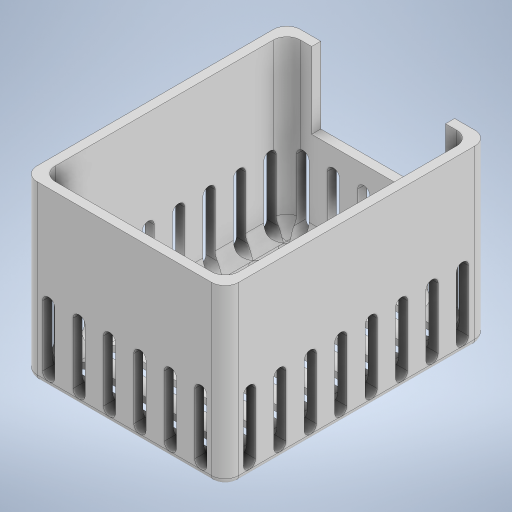
# Autodesk Inventor part: ProtectiveCase
Saved by Autodesk Inventor 2023 (Build 270158000, 158)
## iProperties
Created: 2024-02-01
Part Number: ProtectiveCase
Material: Generic
Document SubType Name: Modeling
Designer: Daniil
Density: 1 g/cm^3
Appearance: Default
Author: Daniil
Autodesk Inventor part; units mm, degrees
ref_plane "YZ Plane" through (0, 0, 0) normal (1, 0, 0) x (0, 1, 0)
ref_plane "XZ Plane" through (0, 0, 0) normal (0, 1, 0) x (-1, 0, 0)
ref_plane "XY Plane" through (0, 0, 0) normal (0, 0, 1) x (1, 0, 0)
sketch "Sketch1" plane through (0, 0, 0) normal (0, 1, 0) x (-1, 0, 0)
  line L0 (0, 0) -> (66.3, 0)
  line L1 (66.3, 0) -> (66.3, -86.6)
  line L2 (66.3, -86.6) -> (0, -86.6)
  line L3 (0, -86.6) -> (0, 0)
  line L4 (63.3, -3) -> (3, -3)
  line L5 (3, -3) -> (3, -83.6)
  line L6 (3, -83.6) -> (63.3, -83.6)
  line L7 (63.3, -83.6) -> (63.3, -3)
  dimension "d0" = 80.6
  dimension "d1" = 60.3
  dimension "d2" = 3
  dimension "d3" = 3
  dimension "d4" = 3
  dimension "d5" = 3
  constraints: 16 end point, 4 parallel, 2 horizontal, 2 perpendicular
  measures "d0" distance between parallel lines of L6 L4
  measures "d1" distance between parallel lines of L5 L7
  measures "d2" distance between parallel lines of L4 L0
  measures "d3" distance between parallel lines of L3 L5
  measures "d4" distance between parallel lines of L1 L7
  measures "d5" distance between parallel lines of L2 L6
extrude "Extrusion1" add sketch "Sketch1" along normal blind 57
sketch "Sketch2" plane through (0, 0, -86.6) normal (0, 0, -1) x (-1, 0, 0)
  line L0 (0, 0) -> (66.3, 0) projected
  line L1 (66.3, 0) -> (66.3, 57) projected
  line L2 (0, 57) -> (66.3, 57) projected
  line L3 (0, 0) -> (0, 57) projected
  line L4 (63.3, 57) -> (3, 57) construction
  line L5 (33.15, 57) -> (33.15, 0) construction
  line L6 (11.15, 57) -> (55.15, 57)
  line L7 (55.15, 57) -> (55.15, 35)
  line L8 (55.15, 35) -> (11.15, 35)
  line L9 (11.15, 35) -> (11.15, 57)
  point P0 (0, 0)
  dimension "d8" = 44
  dimension "d9" = 22
  constraints: 10 end point, 2 midpoint, 2 parallel, 1 horizontal, 1 perpendicular, 1 point on line, 1 other
  measures "d8" distance between parallel lines of L7 L9
  measures "d9" distance between parallel lines of L8 L2
extrude "Extrusion2" cut sketch "Sketch2" against normal blind 57 contours L2 L7 L8 L9
fillet "Fillet1" radius 4.5 8 edges at (-3, 28.5, -3) (-63.3, 28.5, -3) (-63.3, 28.5, -83.6) (-3, 28.5, -83.6) (0, 28.5, -86.6) (-66.3, 28.5, -86.6) (-66.3, 28.5, 0) (0, 28.5, 0)
sketch "Sketch3" plane through (0, 0, 0) normal (0, -1, 0) x (1, 0, 0)
  line L0 (0, -4.5) -> (0, -82.1) projected
  arc A0 (-4.5, -86.6) -> (0, -82.1) centre (-4.5, -82.1) ccw projected
  line L1 (-4.5, -86.6) -> (-61.8, -86.6) projected
  arc A1 (-66.3, -82.1) -> (-61.8, -86.6) centre (-61.8, -82.1) ccw projected
  line L2 (-66.3, -82.1) -> (-66.3, -4.5) projected
  arc A2 (-61.8, 0) -> (-66.3, -4.5) centre (-61.8, -4.5) ccw projected
  line L3 (-61.8, 0) -> (-4.5, 0) projected
  arc A3 (0, -4.5) -> (-4.5, 0) centre (-4.5, -4.5) ccw projected
  point P0 (0, 0)
extrude "Extrusion3" add sketch "Sketch3" against normal blind 2
sketch "Sketch4" plane through (0, 0, -4.5) normal (1, 0, 0) x (0, 0, -1)
  line L0 (-1.5, 2) -> (3, 2) projected
  line L1 (3, 2) -> (-1.5, 2) projected
  line L2 (74.6, 2) -> (3, 2) projected
  line L3 (79.1, 2) -> (74.6, 2) projected
  line L4 (74.6, 2) -> (79.1, 2) projected
  line L5 (3, 2) -> (74.6, 2) projected
  line L6 (-1.5, 57) -> (-1.5, 2) projected
  line L7 (-1.5, 2) -> (-1.5, 57) projected
  line L8 (79.1, 57) -> (79.1, 2) projected
  line L9 (79.1, 57) -> (79.1, 35) projected
  line L10 (79.1, 35) -> (79.1, 57) projected
  line L11 (79.1, 2) -> (79.1, 57) projected
  line L12 (-1.5, 26) -> (79.1, 26) construction
  line L13 (3.5, 24) -> (3.5, 4) construction
  line L14 (1.5, 24) -> (1.5, 4)
  line L15 (5.5, 4) -> (5.5, 24)
  arc A0 (5.5, 24) -> (1.5, 24) centre (3.5, 24) ccw
  arc A1 (1.5, 4) -> (5.5, 4) centre (3.5, 4) ccw
  arc A2 (15.5, 24) -> (11.5, 24) centre (13.5, 24) ccw
  line L16 (11.5, 24) -> (11.5, 4)
  line L17 (15.5, 4) -> (15.5, 24)
  arc A3 (11.5, 4) -> (15.5, 4) centre (13.5, 4) ccw
  arc A4 (25.5, 24) -> (21.5, 24) centre (23.5, 24) ccw
  line L18 (21.5, 24) -> (21.5, 4)
  line L19 (25.5, 4) -> (25.5, 24)
  arc A5 (21.5, 4) -> (25.5, 4) centre (23.5, 4) ccw
  arc A6 (35.5, 24) -> (31.5, 24) centre (33.5, 24) ccw
  line L20 (31.5, 24) -> (31.5, 4)
  line L21 (35.5, 4) -> (35.5, 24)
  arc A7 (31.5, 4) -> (35.5, 4) centre (33.5, 4) ccw
  arc A8 (45.5, 24) -> (41.5, 24) centre (43.5, 24) ccw
  line L22 (41.5, 24) -> (41.5, 4)
  line L23 (45.5, 4) -> (45.5, 24)
  arc A9 (41.5, 4) -> (45.5, 4) centre (43.5, 4) ccw
  arc A10 (55.5, 24) -> (51.5, 24) centre (53.5, 24) ccw
  line L24 (51.5, 24) -> (51.5, 4)
  line L25 (55.5, 4) -> (55.5, 24)
  arc A11 (51.5, 4) -> (55.5, 4) centre (53.5, 4) ccw
  arc A12 (65.5, 24) -> (61.5, 24) centre (63.5, 24) ccw
  line L26 (61.5, 24) -> (61.5, 4)
  line L27 (65.5, 4) -> (65.5, 24)
  arc A13 (61.5, 4) -> (65.5, 4) centre (63.5, 4) ccw
  arc A14 (75.5, 24) -> (71.5, 24) centre (73.5, 24) ccw
  line L28 (71.5, 24) -> (71.5, 4)
  line L29 (75.5, 4) -> (75.5, 24)
  arc A15 (71.5, 4) -> (75.5, 4) centre (73.5, 4) ccw
  point P0 (-4.5, 0)
  point P1 (3.5, 14)
  dimension "d15" = 24
  dimension "d16" = 4
  dimension "d17" = 5
  dimension "d20" = 10
  constraints: 38 end point, 32 point on circle, 16 centre point, 6 tangent, 2 point on line, 1 horizontal, 1 midpoint, 1 parallel, 1 perpendicular, 1 vertical, 70 other
  measures "d15" distance between parallel lines of L2 L12
  measures "d16" distance between parallel lines of L15 L14
  measures "d17" distance between parallel lines of L13 L6
  measures "d20" distance of L13.start A2.centre
sketch "Sketch5" plane through (-11.15, 35, -86.6) normal (0, 0, -1) x (-1, 0, 0)
  line L0 (47.65, -33) -> (52.15, -33) projected
  line L1 (-3.65, -33) -> (47.65, -33) projected
  line L2 (-8.15, -33) -> (-3.65, -33) projected
  line L3 (-3.65, -33) -> (-8.15, -33) projected
  line L4 (47.65, -33) -> (-3.65, -33) projected
  line L5 (52.15, -33) -> (47.65, -33) projected
  line L6 (52.15, 22) -> (52.15, -33) projected
  line L7 (52.15, -33) -> (52.15, 22) projected
  line L8 (-8.15, 22) -> (-8.15, -33) projected
  line L9 (-8.15, -33) -> (-8.15, 22) projected
  line L10 (-8.15, 22) -> (-8.15, -33) construction
  line L11 (-8.15, -9) -> (52.15, -9) construction
  line L12 (-3.15, -11) -> (-3.15, -31) construction
  line L13 (-5.15, -11) -> (-5.15, -31)
  line L14 (-1.15, -31) -> (-1.15, -11)
  arc A0 (-1.15, -11) -> (-5.15, -11) centre (-3.15, -11) ccw
  arc A1 (-5.15, -31) -> (-1.15, -31) centre (-3.15, -31) ccw
  arc A2 (8.85, -11) -> (4.85, -11) centre (6.85, -11) ccw
  line L15 (4.85, -11) -> (4.85, -31)
  line L16 (8.85, -31) -> (8.85, -11)
  arc A3 (4.85, -31) -> (8.85, -31) centre (6.85, -31) ccw
  arc A4 (18.85, -11) -> (14.85, -11) centre (16.85, -11) ccw
  line L17 (14.85, -11) -> (14.85, -31)
  line L18 (18.85, -31) -> (18.85, -11)
  arc A5 (14.85, -31) -> (18.85, -31) centre (16.85, -31) ccw
  arc A6 (28.85, -11) -> (24.85, -11) centre (26.85, -11) ccw
  line L19 (24.85, -11) -> (24.85, -31)
  line L20 (28.85, -31) -> (28.85, -11)
  arc A7 (24.85, -31) -> (28.85, -31) centre (26.85, -31) ccw
  arc A8 (38.85, -11) -> (34.85, -11) centre (36.85, -11) ccw
  line L21 (34.85, -11) -> (34.85, -31)
  line L22 (38.85, -31) -> (38.85, -11)
  arc A9 (34.85, -31) -> (38.85, -31) centre (36.85, -31) ccw
  arc A10 (48.85, -11) -> (44.85, -11) centre (46.85, -11) ccw
  line L23 (44.85, -11) -> (44.85, -31)
  line L24 (48.85, -31) -> (48.85, -11)
  arc A11 (44.85, -31) -> (48.85, -31) centre (46.85, -31) ccw
  point P0 (-11.15, -35)
  point P1 (-8.15, -33)
  point P2 (-8.15, -33)
  point P3 (-8.15, -33)
  point P4 (-8.15, -33)
  point P5 (-8.15, -33)
  point P6 (-8.15, -9.3297)
  point P7 (-8.15, -11)
  point P8 (-8.15, -31)
  point P9 (-8.15, -31)
  point P10 (-8.15, -11)
  point P11 (-8.15, -11)
  point P12 (-8.15, -31)
  point P13 (-8.15, -33)
  point P14 (-8.15, -31)
  point P15 (-8.15, -11)
  point P16 (-8.15, -11)
  point P17 (-8.15, -31)
  point P18 (-8.15, -33)
  point P19 (-8.15, -31)
  point P20 (-8.15, -11)
  point P21 (-8.15, -11)
  point P22 (-8.15, -31)
  point P23 (-8.15, -33)
  point P24 (-8.15, -31)
  point P25 (-8.15, -11)
  point P26 (-8.15, -11)
  point P27 (-8.15, -31)
  point P28 (-8.15, -33)
  point P29 (-8.15, -31)
  point P30 (-8.15, -11)
  point P31 (-8.15, -11)
  point P32 (-8.15, -31)
  point P33 (-8.15, -33)
  point P34 (-8.15, -31)
  point P35 (-8.15, -11)
  point P36 (-8.15, -11)
  point P37 (-8.15, -31)
  point P38 (-8.15, -31)
  point P39 (-8.15, -11)
  point P40 (-8.15, -9.0635)
  point P41 (-3.15, -21)
  dimension "d27" = 24
  dimension "d28" = 4
  dimension "d29" = 5
  dimension "d32" = 10
  constraints: 30 end point, 24 point on circle, 12 centre point, 6 tangent, 2 horizontal, 1 midpoint, 1 parallel, 1 vertical, 52 other
  measures "d27" distance between parallel lines of L1 L11
  measures "d28" distance between parallel lines of L14 L13
  measures "d32" distance of L12.start A2.centre
sketch "Sketch6" plane through (0, 2, 0) normal (0, 1, 0) x (1, 0, 0)
  line L0 (-7.5, 3) -> (-58.8, 3) projected
  arc A0 (-7.5, 3) -> (-3, 7.5) centre (-7.5, 7.5) ccw projected
  line L1 (-3, 79.1) -> (-3, 7.5) projected
  arc A1 (-3, 79.1) -> (-7.5, 83.6) centre (-7.5, 79.1) ccw projected
  line L2 (-58.8, 83.6) -> (-7.5, 83.6) projected
  arc A2 (-58.8, 83.6) -> (-63.3, 79.1) centre (-58.8, 79.1) ccw projected
  line L3 (-63.3, 7.5) -> (-63.3, 79.1) projected
  arc A3 (-63.3, 7.5) -> (-58.8, 3) centre (-58.8, 7.5) ccw projected
  line L4 (-7.5, 7.5) -> (-58.8, 7.5) construction
  line L5 (-58.8, 7.5) -> (-58.8, 79.1)
  line L6 (-58.8, 79.1) -> (-7.5, 79.1) construction
  line L7 (-7.5, 79.1) -> (-7.5, 7.5) construction
  line L8 (-9.5, 9.5) -> (-56.8, 9.5) construction
  line L9 (-9.5, 11.5) -> (-56.8, 11.5)
  line L10 (-56.8, 7.5) -> (-9.5, 7.5)
  arc A4 (-9.5, 7.5) -> (-9.5, 11.5) centre (-9.5, 9.5) ccw
  arc A5 (-56.8, 11.5) -> (-56.8, 7.5) centre (-56.8, 9.5) ccw
  arc A6 (-9.5, 17.15) -> (-9.5, 21.15) centre (-9.5, 19.15) ccw
  line L11 (-56.8, 17.15) -> (-9.5, 17.15)
  line L12 (-9.5, 21.15) -> (-56.8, 21.15)
  arc A7 (-56.8, 21.15) -> (-56.8, 17.15) centre (-56.8, 19.15) ccw
  arc A8 (-9.5, 26.8) -> (-9.5, 30.8) centre (-9.5, 28.8) ccw
  line L13 (-56.8, 26.8) -> (-9.5, 26.8)
  line L14 (-9.5, 30.8) -> (-56.8, 30.8)
  arc A9 (-56.8, 30.8) -> (-56.8, 26.8) centre (-56.8, 28.8) ccw
  arc A10 (-9.5, 36.45) -> (-9.5, 40.45) centre (-9.5, 38.45) ccw
  line L15 (-56.8, 36.45) -> (-9.5, 36.45)
  line L16 (-9.5, 40.45) -> (-56.8, 40.45)
  arc A11 (-56.8, 40.45) -> (-56.8, 36.45) centre (-56.8, 38.45) ccw
  arc A12 (-9.5, 46.1) -> (-9.5, 50.1) centre (-9.5, 48.1) ccw
  line L17 (-56.8, 46.1) -> (-9.5, 46.1)
  line L18 (-9.5, 50.1) -> (-56.8, 50.1)
  arc A13 (-56.8, 50.1) -> (-56.8, 46.1) centre (-56.8, 48.1) ccw
  arc A14 (-9.5, 55.75) -> (-9.5, 59.75) centre (-9.5, 57.75) ccw
  line L19 (-56.8, 55.75) -> (-9.5, 55.75)
  line L20 (-9.5, 59.75) -> (-56.8, 59.75)
  arc A15 (-56.8, 59.75) -> (-56.8, 55.75) centre (-56.8, 57.75) ccw
  arc A16 (-9.5, 65.4) -> (-9.5, 69.4) centre (-9.5, 67.4) ccw
  line L21 (-56.8, 65.4) -> (-9.5, 65.4)
  line L22 (-9.5, 69.4) -> (-56.8, 69.4)
  arc A17 (-56.8, 69.4) -> (-56.8, 65.4) centre (-56.8, 67.4) ccw
  arc A18 (-9.5, 75.05) -> (-9.5, 79.05) centre (-9.5, 77.05) ccw
  line L23 (-56.8, 75.05) -> (-9.5, 75.05)
  line L24 (-9.5, 79.05) -> (-56.8, 79.05)
  arc A19 (-56.8, 79.05) -> (-56.8, 75.05) centre (-56.8, 77.05) ccw
  point P0 (0, 0)
  point P1 (-33.15, 9.5)
  dimension "d39" = 4
  dimension "d42" = 9.65
  constraints: 44 end point, 32 point on circle, 16 centre point, 6 tangent, 4 parallel, 1 collinear, 1 horizontal, 1 midpoint, 1 perpendicular, 1 vertical, 70 other
  measures "d39" distance between parallel lines of L9 L10
  measures "d42" distance of L8.start A6.centre
extrude "Extrusion6" cut sketch "Sketch6" against normal blind 100 contours A19 L24 A18 L23 | A17 L22 A16 L21 | A15 L20 A14 L19 | A13 L18 A12 L17 | A11 L16 A10 L15 | A9 L14 A8 L13 | A7 L12 A6 L11 | A5 L9 A4 L10
fillet "Fillet2" radius 4.5 8 edges at (-3, 2, -43.3) (-4.318, 2, -4.318) (-33.15, 2, -3) (-61.982, 2, -4.318) (-63.3, 2, -43.3) (-61.982, 2, -82.282) (-33.15, 2, -83.6) (-4.318, 2, -82.282)
extrude "Extrusion7" cut sketch "Sketch4" against normal blind 100
extrude "Extrusion8" cut sketch "Sketch5" against normal blind 100
fillet "Fillet3" radius 2 8 edges at (-64.982, 0, -85.282) (-66.3, 0, -43.3) (-64.982, 0, -1.318) (-33.15, 0, 0) (-1.318, 0, -1.318) (0, 0, -43.3) (-1.318, 0, -85.282) (-33.15, 0, -86.6)
sketch "Sketch7" plane through (-11.15, 35, -86.6) normal (0, 0, -1) x (-1, 0, 0)
  line L0 (-3.15, -33) -> (-6.65, -33) projected
  arc A0 (-5.15, -31) -> (-3.15, -33) centre (-3.15, -31) ccw projected
  line L1 (-5.15, -31) -> (-5.15, -11) projected
  arc A1 (-1.15, -11) -> (-5.15, -11) centre (-3.15, -11) ccw projected
  line L2 (-1.15, -11) -> (-1.15, -31) projected
  arc A2 (-3.15, -33) -> (-1.15, -31) centre (-3.15, -31) ccw projected
  line L3 (6.85, -33) -> (-3.15, -33) projected
  arc A3 (4.85, -31) -> (6.85, -33) centre (6.85, -31) ccw projected
  line L4 (4.85, -31) -> (4.85, -11) projected
  arc A4 (8.85, -11) -> (4.85, -11) centre (6.85, -11) ccw projected
  line L5 (8.85, -11) -> (8.85, -31) projected
  arc A5 (6.85, -33) -> (8.85, -31) centre (6.85, -31) ccw projected
  line L6 (16.85, -33) -> (6.85, -33) projected
  arc A6 (14.85, -31) -> (16.85, -33) centre (16.85, -31) ccw projected
  line L7 (14.85, -31) -> (14.85, -11) projected
  arc A7 (18.85, -11) -> (14.85, -11) centre (16.85, -11) ccw projected
  line L8 (18.85, -11) -> (18.85, -31) projected
  arc A8 (16.85, -33) -> (18.85, -31) centre (16.85, -31) ccw projected
  line L9 (26.85, -33) -> (16.85, -33) projected
  arc A9 (24.85, -31) -> (26.85, -33) centre (26.85, -31) ccw projected
  line L10 (24.85, -31) -> (24.85, -11) projected
  arc A10 (28.85, -11) -> (24.85, -11) centre (26.85, -11) ccw projected
  line L11 (28.85, -11) -> (28.85, -31) projected
  arc A11 (26.85, -33) -> (28.85, -31) centre (26.85, -31) ccw projected
  line L12 (36.85, -33) -> (26.85, -33) projected
  arc A12 (34.85, -31) -> (36.85, -33) centre (36.85, -31) ccw projected
  line L13 (34.85, -31) -> (34.85, -11) projected
  arc A13 (38.85, -11) -> (34.85, -11) centre (36.85, -11) ccw projected
  line L14 (38.85, -11) -> (38.85, -31) projected
  arc A14 (36.85, -33) -> (38.85, -31) centre (36.85, -31) ccw projected
  line L15 (46.85, -33) -> (36.85, -33) projected
  arc A15 (44.85, -31) -> (46.85, -33) centre (46.85, -31) ccw projected
  line L16 (44.85, -31) -> (44.85, -11) projected
  arc A16 (48.85, -11) -> (44.85, -11) centre (46.85, -11) ccw projected
  line L17 (48.85, -11) -> (48.85, -31) projected
  arc A17 (46.85, -33) -> (48.85, -31) centre (46.85, -31) ccw projected
  line L18 (50.65, -33) -> (46.85, -33) projected
  line L19 (50.65, 22) -> (50.65, -33) projected
  line L20 (44, 22) -> (50.65, 22) projected
  line L21 (44, 22) -> (44, 0) projected
  line L22 (44, 0) -> (0, 0) projected
  line L23 (0, 0) -> (0, 22) projected
  line L24 (-6.65, 22) -> (0, 22) projected
  line L25 (-6.65, -33) -> (-6.65, 22) projected
  line L26 (0, 0) -> (44, 0)
  line L27 (44, 0) -> (44, -3)
  line L28 (44, -3) -> (0, -3)
  line L29 (0, -3) -> (0, 0)
  point P0 (-11.15, -35)
  dimension "d55" = 25
  constraints: 8 end point, 2 parallel, 1 horizontal, 1 perpendicular
  measures "d55" distance between parallel lines of L28 L24
extrude "Extrusion9" cut sketch "Sketch7" against normal blind 10 contours L22 L27 L28 L29
body "Solid1"
